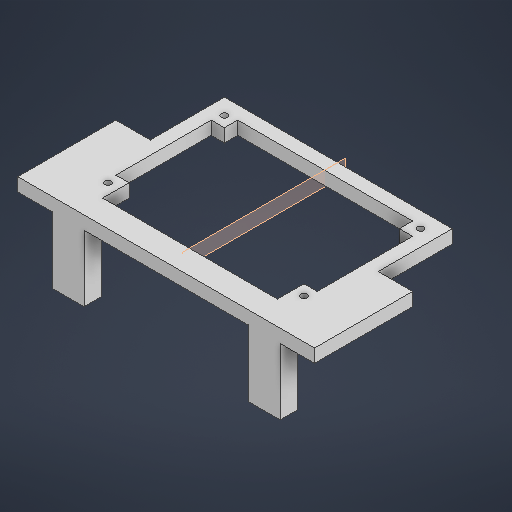
# Autodesk Inventor part: PCB_Housing_01_001_V2
Saved by Autodesk Inventor 2026.2 (Build 302298000, 298)
## iProperties
Created: 2026-02-04
Part Number: PCB_Housing_01_001_V2
Material: Generic
Document SubType Name: Modeling
Designer: vckot
Density: 1 g/cm^3
Appearance: Default
Author: vckot
Autodesk Inventor part; units mm, degrees
ref_plane "YZ Plane" through (0, 0, 0) normal (1, 0, 0) x (0, 1, 0)
ref_plane "XZ Plane" through (0, 0, 0) normal (0, 1, 0) x (-1, 0, 0)
ref_plane "XY Plane" through (0, 0, 0) normal (0, 0, 1) x (1, 0, 0)
sketch "Sketch1" plane through (0, 0, 0) normal (0, 1, 0) x (-1, 0, 0)
  line L0 (-37, 22) -> (37, 22) construction
  line L1 (37, 22) -> (37, -22) construction
  line L2 (37, -22) -> (-37, -22) construction
  line L3 (-37, -22) -> (-37, 22) construction
  line L4 (-37, 22) -> (37, -22) construction
  line L5 (37, 22) -> (-37, -22) construction
  line L6 (-47, 32) -> (47, 32) construction
  line L7 (47, 32) -> (47, -32) construction
  line L8 (47, -32) -> (-47, -32) construction
  line L9 (-47, -32) -> (-47, 32) construction
  line L10 (-47, 32) -> (47, -32) construction
  line L11 (47, 32) -> (-47, -32) construction
  line L12 (31, 16) -> (43, 16)
  line L13 (43, 16) -> (43, 28)
  line L14 (43, 28) -> (31, 28)
  line L15 (31, 28) -> (31, 16)
  line L16 (31, 16) -> (43, 28) construction
  line L17 (43, 16) -> (31, 28) construction
  line L18 (47, 0) -> (-47, 0) construction
  line L19 (0, 32) -> (0, -32) construction
  line L20 (37, -22) -> (-37, 22) construction
  line L21 (47, -32) -> (-47, 32) construction
  line L22 (31, -16) -> (43, -16)
  line L23 (43, -16) -> (43, -28)
  line L24 (43, -28) -> (31, -28)
  line L25 (31, -28) -> (31, -16)
  line L26 (31, -16) -> (43, -28) construction
  line L27 (43, -16) -> (31, -28) construction
  line L28 (-31, 16) -> (-43, 16)
  line L29 (-43, 16) -> (-43, 28)
  line L30 (-43, 28) -> (-31, 28)
  line L31 (-31, 28) -> (-31, 16)
  line L32 (-31, -16) -> (-43, -16)
  line L33 (-31, -28) -> (-31, -16)
  line L34 (-43, -28) -> (-31, -28)
  line L35 (-43, -16) -> (-43, -28)
  line L36 (43, 28) -> (-43, 28)
  line L37 (-43, 28) -> (-43, -28)
  line L38 (-43, -28) -> (43, -28)
  line L39 (43, -28) -> (43, 28)
  point P0 (0, 0)
  dimension "d0" = 74
  dimension "d1" = 44
  dimension "d2" = 10
  dimension "d3" = 10
  dimension "d4" = 12
  dimension "d5" = 12
  constraints: 80 end point, 12 symmetric about line, 10 midpoint, 8 parallel, 4 horizontal, 4 perpendicular
  measures "d0" distance of L1.end L2.end
  measures "d1" distance of L0.end L1.end
  measures "d2" distance between parallel lines of L8 L2
  measures "d3" distance between parallel lines of L7 L1
  measures "d4" distance of L14.end L13.end
  measures "d5" distance of L13.end L12.end
extrude "Extrusion1" add sketch "Sketch1" against normal blind 5
extrude "Extrusion2" add sketch "Sketch1" against normal blind 30 contours L15 L14 L13 L12 | L23 L24 L25 L22 | L31 L28 L29 L30 | L34 L35 L32 L33
hole "Hole2" at (-37, 0, 22) at (-37, 0, -22) at (37, 0, -22) at (37, 0, 22) direction (0, -1, 0) diameter 2.4 depth 8 tip angle 118 clearance for "Flat Head Machine Screw" size "M2" standard "Ansi Metric M Profile"
sketch "Sketch4" plane through (0, -30, 0) normal (0, -1, 0) x (1, 0, 0)
  line L0 (31, 28) -> (-31, 28) projected
  line L1 (-43, 16) -> (-31, 16) projected
  line L2 (31, 28) -> (-31, 28)
  line L3 (-31, 28) -> (-31, 16)
  line L4 (-31, 16) -> (31, 16)
  line L5 (31, 16) -> (31, 28)
  line L6 (43, -28) -> (-43, -28) projected
  line L7 (-43, -16) -> (-31, -16) projected
  line L8 (31, -28) -> (-31, -28)
  line L9 (-31, -28) -> (-31, -16)
  line L10 (-31, -16) -> (31, -16)
  line L11 (31, -16) -> (31, -28)
  point P0 (0, 0)
  constraints: 16 end point, 4 parallel, 2 horizontal, 2 perpendicular, 2 point on line
extrude "Extrusion3" add sketch "Sketch4" against normal blind 10
sketch "Sketch5" plane through (0, -30, 0) normal (0, -1, 0) x (1, 0, 0)
  circle A0 centre (37, 22) radius 1.2 projected
  circle A1 centre (-37, 22) radius 1.2 projected
  circle A2 centre (-37, -22) radius 1.2 projected
  circle A3 centre (37, -22) radius 1.2 projected
  point P0 (0, 0)
hole "Hole3" at (37, -30, 22) at (-37, -30, 22) at (-37, -30, -22) at (37, -30, -22) direction (0, 1, 0) diameter 5.35 depth 10 tip angle 118
sketch "Sketch6" plane through (-43, 0, 28) normal (0, 0, 1) x (1, 0, 0)
  line L0 (0, -5) -> (12, -5) projected
  line L1 (86, -30) -> (0, -30) projected
  line L2 (0, -5) -> (86, -5)
  line L3 (86, -5) -> (86, -30)
  line L4 (86, -30) -> (0, -30)
  line L5 (0, -30) -> (0, -5)
  point P0 (43, 0)
  constraints: 8 end point, 2 parallel, 1 horizontal, 1 perpendicular
extrude "Extrusion4" cut sketch "Sketch6" against normal through all
sketch "Sketch7" plane through (43, 0, 28) normal (1, 0, 0) x (0, 0, -1)
  line L0 (0, 0) -> (0, -5) projected
  line L1 (56, -5) -> (0, -5) projected
  line L2 (0, 0) -> (28, 0)
  line L3 (28, 0) -> (28, -5)
  line L4 (28, -5) -> (0, -5)
  line L5 (0, -5) -> (0, 0)
  constraints: 8 end point, 2 parallel, 1 horizontal, 1 midpoint, 1 perpendicular
extrude "Extrusion5" add sketch "Sketch7" along normal blind 13
ref_plane "Work Plane1" through (0, -5, -28) normal (1, 0, 0) x (0, 0, -1)
mirror "Mirror1" about plane through (0, -5, -28) normal (1, 0, 0) of "Extrusion5"
thicken "Thicken1" operation add thickness 9 both sides no extend neighbours no toward (0, 0, 1) faces at (18.6667, -1.6667, 28)
sketch "Sketch8" plane through (0, -5, 0) normal (0, -1, 0) x (1, 0, 0)
  line L0 (43.815, 30.008) -> (-43.815, 30.008) projected
  line L1 (-56, 37) -> (56, 37) projected
  line L2 (-43, 37) -> (-31, 37)
  line L3 (-31, 37) -> (-31, 30.5)
  line L4 (-31, 30.5) -> (-43, 30.5)
  line L5 (-43, 30.5) -> (-43, 37)
  circle A0 centre (-37, 22) radius 1.2 projected
  circle A1 centre (37, 22) radius 1.2 projected
  line L6 (0, 37) -> (0, 11.1559) construction
  line L7 (-43.815, 30.008) -> (43.815, 30.008)
  line L8 (43, 37) -> (31, 37)
  line L9 (31, 37) -> (31, 30.5)
  line L10 (31, 30.5) -> (43, 30.5)
  line L11 (43, 30.5) -> (43, 37)
  point P0 (0, 0)
  point P1 (-37, 30.5)
  point P2 (37, 30.5)
  dimension "d44" = 12
  dimension "d45" = 6.5
  constraints: 20 end point, 7 symmetric about line, 2 midpoint, 2 parallel, 1 horizontal, 1 perpendicular, 1 point on line, 1 vertical, 1 vertical alignment
  measures "d44" distance of L3.end L4.end
  measures "d45" distance of L2.end L3.end
extrude "Extrusion6" add sketch "Sketch8" along normal blind 25 contours L1 L3 L4 L5 | L1 L11 L10 L9
sketch "Sketch9" plane through (0, -30, 0) normal (0, -1, 0) x (1, 0, 0)
  line L0 (43, 30.5) -> (43, 37) projected
  line L1 (-43, 37) -> (-43, 30.5) projected
  line L2 (-31, 37) -> (-43, 37) projected
  point P0 (0, 0)
  point P1 (-37, 33.75)
  point P2 (37, 33.75)
  dimension "d48" = 6
  dimension "d49" = 6
  dimension "d50" = 3.25
  constraints: 1 horizontal alignment
  measures "d48" distance from line of L0 point (37, 33.75)
  measures "d49" distance from line of L1 point (-37, 33.75)
  measures "d50" distance from line of L2 point (-37, 33.75)
hole "Hole4" at (-37, -30, 33.75) at (37, -30, 33.75) direction (0, 1, 0) diameter 5.35 depth 10 tip angle 118
sketch "Sketch10" plane through (0, 0, 0) normal (0, 1, 0) x (1, 0, 0)
  line L0 (-31, 16) -> (-43, 16) projected
  line L1 (-31, 28) -> (-31, 16) projected
  line L2 (-31, -16) -> (-43, -16) projected
  line L3 (-31, -28) -> (-31, -16) projected
  line L4 (31, -28) -> (31, -16) projected
  line L5 (31, -16) -> (43, -16) projected
  line L6 (31, 16) -> (43, 16) projected
  line L7 (31, 28) -> (31, 16) projected
  line L8 (-33, 23) -> (33, 23)
  line L9 (38, 18) -> (38, -18)
  line L10 (-33, -28) -> (33, -28)
  line L11 (-38, -18) -> (-38, 18)
  line L12 (-43, 28) -> (-43, 0) projected
  line L13 (43, 28) -> (-43, 28) projected
  line L14 (43, 0) -> (43, 28) projected
  line L15 (-33, -28) -> (-33, -18)
  line L16 (-33, -18) -> (-43, -18)
  line L17 (43, -18) -> (33, -18)
  line L18 (33, -18) -> (33, -28)
  line L19 (33, 28) -> (33, 18)
  line L20 (33, 18) -> (43, 18)
  line L21 (-33, 28) -> (-33, 18)
  line L22 (-33, 18) -> (-43, 18)
  point P0 (0, 0)
  point P1 (-31, 23)
  point P2 (31, 23)
  point P3 (38, 16)
  point P4 (38, -16)
  point P5 (-31, -28)
  point P6 (31, -28)
  point P7 (-38, -16)
  point P8 (-38, 16)
  dimension "d58" = 5
  dimension "d59" = 5
  dimension "d60" = 5
  dimension "d61" = 0
  dimension "d66" = 2
  dimension "d67" = 2
  dimension "d68" = 2
  dimension "d69" = 2
  constraints: 24 end point, 16 point on line, 6 midpoint, 4 perpendicular, 4 other
  measures "d58" distance between parallel lines of L12 L11
  measures "d59" distance between parallel lines of L13 L8
  measures "d60" distance between parallel lines of L14 L9
  measures "d61" distance from line of L4.start L10
  measures "d66" distance between parallel lines of L3 L15
  measures "d67" distance between parallel lines of L5 L17
  measures "d68" distance between parallel lines of L7 L19
  measures "d69" distance between parallel lines of L1 L21
extrude "Extrusion7" cut sketch "Sketch10" against normal through all contours L1 L8 L7 L6 L9 L5 L4 L10 L3 L2 L11 L0 | L0 L11 L22 L21 L8 L1 | L2 L3 L10 L15 L16 L11 | L8 L19 L20 L9 L6 L7 | L4 L5 L9 L17 L18 L10
body "Solid1"
